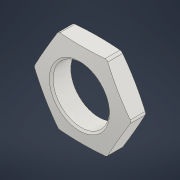
# Autodesk Inventor part: ecrou
Saved by Autodesk Inventor 2022.1 (Build 261234020, 234B)
## iProperties
Created: 2021-12-02
Part Number: ecrou
Material: Generic
Document SubType Name: Modeling
Designer: PaulT
Density: 1 g/cm^3
Appearance: Steel
Author: PaulT
Autodesk Inventor part; units mm, degrees
ref_plane "YZ Plane" through (0, 0, 0) normal (1, 0, 0) x (0, 1, 0)
ref_plane "XZ Plane" through (0, 0, 0) normal (0, 1, 0) x (-1, 0, 0)
ref_plane "XY Plane" through (0, 0, 0) normal (0, 0, 1) x (1, 0, 0)
sketch "Sketch1" plane through (0, 0, 0) normal (0, 0, 1) x (1, 0, 0)
  line L0 (4.6765, 0) -> (2.3383, -4.05)
  line L1 (2.3383, -4.05) -> (-2.3383, -4.05)
  line L2 (-2.3383, -4.05) -> (-4.6765, 0)
  line L3 (-4.6765, 0) -> (-2.3383, 4.05)
  line L4 (-2.3383, 4.05) -> (2.3383, 4.05)
  line L5 (2.3383, 4.05) -> (4.6765, 0)
  point P0 (0, 0)
  point P1 (0, 0)
  dimension "d0" = 8.1
  constraints: 12 end point, 1 coincident, 13 other
  measures "d0" distance between parallel lines of L1 L4
extrude "Extrusion1" add sketch "Sketch1" along normal mid plane 2.1
sketch "Sketch2" plane through (0, 0, -1.05) normal (0, 0, -1) x (1, 0, 0)
  circle A0 centre (0, 0) radius 2.7
  dimension "d3" = 5.4
  constraints: 1 centre point, 1 coincident
  measures "d3" diameter of A0
extrude "Extrusion2" cut sketch "Sketch2" against normal blind 2.1
fillet "Fillet2" radius 0.3 6 edges at (-2.3383, 4.05, 0) (2.3383, 4.05, 0) (-4.6765, 0, 0) (-2.3383, -4.05, 0) (2.3383, -4.05, 0) (4.6765, 0, 0)
sketch "Sketch4" plane through (0, 0, 0) normal (1, 0, 0) x (0, 1, 0)
  line L0 (2.7, 1.05) -> (5, 1.05)
  line L1 (5, 1.05) -> (5, 0.6444)
  line L2 (5, 0.6444) -> (2.7, 1.05)
  line L3 (-2.7, 1.05) -> (2.7, 1.05) projected
  line L4 (0, 6.5189) -> (0, -6.6611) construction
  line L5 (0, -9.297) -> (0, 9.1548) projected
  point P0 (0, 0)
  point P1 (5, 0.8472)
  dimension "d26" = 5
  dimension "d27" = 10
  constraints: 8 end point, 1 collinear, 1 horizontal, 1 midpoint, 1 perpendicular, 1 vertical
  measures "d26" horizontal distance of point (0, 0) point (5, 0.847)
  measures "d27" angle of L0 L2
revolve "Revolution2" cut sketch "Sketch4" angle 360 about axis through (0, 0, 6.5189) along (0, 0, -1)
mirror "Mirror2" about plane through (0, 0, 0) normal (0, 0, 1) of "Revolution2"
chamfer "Chamfer4" distance 0.2 angle 45 4 edges at (-1.9092, -1.9092, 1.05) (1.9092, 1.9092, 1.05) (-1.9092, -1.9092, -1.05) (1.9092, 1.9092, -1.05)
body "Solid1"
